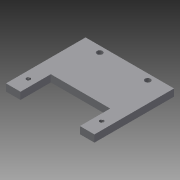
# Autodesk Inventor part: Servo Mount1
Saved by Autodesk Inventor 2013 (Build 170138000, 138)
## iProperties
Created: 2012-10-28
Part Number: Servo Mount1
Material: Generic
Document SubType Name: Modeling
Designer: uqgtayle
Density: 1 g/cm^3
Author: uqgtayle
Autodesk Inventor part; units mm, degrees
ref_plane "YZ Plane" through (0, 0, 0) normal (1, 0, 0) x (0, 1, 0)
ref_plane "XZ Plane" through (0, 0, 0) normal (0, 1, 0) x (-1, 0, 0)
ref_plane "XY Plane" through (0, 0, 0) normal (0, 0, 1) x (1, 0, 0)
sketch "Sketch1" plane through (0, 0, 0) normal (0, 0, 1) x (1, 0, 0)
  line L0 (0, 0) -> (35, 0)
  line L1 (35, 0) -> (35, -31.5)
  line L2 (35, -31.5) -> (0, -31.5)
  line L3 (0, -31.5) -> (0, 0)
  dimension "d0" = 31.5
  dimension "d1" = 35
  constraints: 8 end point, 2 parallel, 1 horizontal, 1 perpendicular
  measures "d0" distance of L2.end L0.start
  measures "d1" distance of L0.start L0.end
extrude "Extrusion1" add sketch "Sketch1" against normal blind 2.8
sketch "Sketch2" plane through (0, 0, 0) normal (0, 0, 1) x (1, 0, 0)
  line L0 (35, -31.5) -> (0, -31.5) projected
  line L1 (5.75, -37.2591) -> (29.25, -37.2591)
  line L2 (29.25, -37.2591) -> (29.25, -19.5)
  line L3 (29.25, -19.5) -> (5.75, -19.5)
  line L4 (5.75, -19.5) -> (5.75, -37.2591)
  point P0 (17.5, -19.5)
  point P1 (17.5, -31.5)
  dimension "d4" = 12
  dimension "d5" = 23.5
  constraints: 8 end point, 2 midpoint, 2 parallel, 1 horizontal, 1 perpendicular, 1 vertical alignment
  measures "d4" distance between parallel lines of L3 L0
  measures "d5" distance of L2.end L3.end
extrude "Extrusion2" cut sketch "Sketch2" against normal through all
sketch "Sketch3" plane through (0, 0, 0) normal (0, 0, 1) x (1, 0, 0)
  line L0 (0, 0) -> (35, 0) projected
  line L1 (0, -31.5) -> (0, 0) projected
  point P0 (8, -2.4)
  point P1 (27, -2.4)
  dimension "d8" = 8
  dimension "d9" = 19
  dimension "d10" = 2.4
  measures "d8" distance from line of point (8, -2.4) L1
  measures "d9" distance of point (27, -2.4) point (8, -2.4)
  measures "d10" distance from line of L0 point (8, -2.4)
hole "Hole1" at (8, -2.4, 0) at (27, -2.4, 0) direction (0, 0, -1) diameter 2.2 end through all
sketch "Sketch4" plane through (0, 0, 0) normal (0, 0, 1) x (1, 0, 0)
  line L0 (29.25, -19.5) -> (29.25, -31.5) projected
  line L1 (5.75, -31.5) -> (0, -31.5) projected
  line L2 (5.75, -31.5) -> (5.75, -19.5) projected
  point P0 (2.875, -25.5)
  point P1 (31.875, -25.5)
  point P2 (5.75, -25.5)
  point P3 (29.25, -25.5)
  point P4 (2.875, -31.5)
  constraints: 3 horizontal alignment, 3 midpoint, 1 vertical alignment
hole "Hole2" at (2.875, -25.5, 0) at (31.875, -25.5, 0) direction (0, 0, -1) diameter 1.567 end through all thread size "M2x0.4" class "6H" standard "ISO Metric profile"
body "Solid1"
